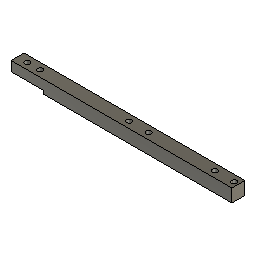
Horizontal_V11 (Autodesk Fusion 360 archive; units mm, degrees)
design "MainArm_Square"
description: .5"x.5"x8.5"
Autodesk Fusion 360 part; units mm, degrees
note: some values were not read from the file. Set by a fixed rule: the direction of a hole.
sketch "LeftEnd" plane through (0, 0, 0) normal (1, 0, 0) x (0, 1, 0) in component "MainArm_Square"
  line L0 (-6.35, -6.35) -> (6.35, -6.35)
  line L1 (6.35, -6.35) -> (6.35, 6.35)
  line L2 (6.35, 6.35) -> (-6.35, 6.35)
  line L3 (-6.35, 6.35) -> (-6.35, -6.35)
  line L4 (-6.35, -6.35) -> (6.35, 6.35) construction
  line L5 (6.35, -6.35) -> (-6.35, 6.35) construction
  dimension "d1" = 12.7
  dimension "d2" = 12.7
  constraint horizontal L0
  constraint perpendicular L0 L1
  constraint parallel L0 L2
  constraint parallel L1 L3
  constraint coincident L4 origin
  constraint coincident L5 origin
  measures "d1" distance of L1.end L2.end
  measures "d2" distance of L0.end L1.end
sketch "Top" plane through (0, 0, 0) normal (0, 0, 1) x (1, 0, 0) in component "MainArm_Square"
  line L0 (107.95, -6.35) -> (-107.95, -6.35)
  line L1 (-107.95, -6.35) -> (-107.95, 6.35)
  line L2 (-107.95, 6.35) -> (107.95, 6.35)
  line L3 (107.95, 6.35) -> (107.95, -6.35)
  line L4 (107.95, -6.35) -> (-107.95, 6.35) construction
  line L5 (-107.95, -6.35) -> (107.95, 6.35) construction
  circle A0 centre (104.013, 0) radius 2.4892
  circle A1 centre (84.963, 0) radius 2.4892
  circle A2 centre (-98.425, 0) radius 2.4892
  circle A3 centre (-85.725, 0) radius 2.4892
  line L6 (-76.073, 6.35) -> (-76.073, -6.35)
  circle A4 centre (1.143, 0) radius 2.4892
  circle A5 centre (20.193, 0) radius 2.4892
  dimension "d3" = 215.9
  dimension "d4" = 12.7
  dimension "d5" = 4.9784
  dimension "d6" = 4.9784
  dimension "d7" = 3.937
  dimension "d8" = 19.05
  dimension "d9" = 4.9784
  dimension "d10" = 4.9784
  dimension "d11" = 85.725
  dimension "d12" = 12.7
  dimension "d15" = 31.877
  dimension "d19" = 4.9784
  dimension "d20" = 4.9784
  dimension "d21" = 87.757
  dimension "d23" = 19.05
  constraint horizontal L0
  constraint perpendicular L0 L1
  constraint parallel L0 L2
  constraint parallel L1 L3
  constraint coincident L4 origin
  constraint coincident L5 origin
  constraint horizontal origin A0.centre
  constraint horizontal A0.centre A1.centre
  constraint horizontal origin A3.centre
  constraint horizontal A2.centre A3.centre
  constraint coincident L2 L6.start
  constraint coincident L0 L6.end
  constraint horizontal origin A4.centre
  constraint horizontal origin A5.centre
  measures "d3" distance of L1.end L2.end
  measures "d4" distance of L0.end L1.end
  measures "d5" diameter of A0
  measures "d6" diameter of A1
  measures "d7" distance of L3 A0.centre
  measures "d8" distance of A0.centre A1.centre
  measures "d9" diameter of A2
  measures "d10" diameter of A3
  measures "d11" distance of A3.centre origin
  measures "d12" distance of A2.centre A3.centre
  measures "d15" distance of L1 L6
  measures "d19" diameter of A4
  measures "d20" diameter of A5
  measures "d21" distance of L3 A5.centre
  measures "d23" distance of A4.centre A5.centre
extrude "Extrude1" add sketch "Top" along normal mid plane 12.7 in component "MainArm_Square"
extrude "Extrude2" cut sketch "Top" along normal blind 3.2614 from surface at -6.35 contours L0 L1 L2 L6 in component "MainArm_Square"
component "MainArm_Square" placed x (1, 0, 0) y (0, 1, 0) z (0, 0, 1) at (0, 0, 0)
equation "d5 = d6"
equation "d10 = d9"
equation "d19 = d6"
equation "d20 = d6"

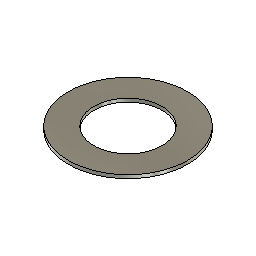
design "Washer_M4x7x0.2"
description: Bearing Washer: M4X7X0.2
Autodesk Fusion 360 part; units mm, degrees
sketch "Sketch1" plane through (0, 0, 0) normal (0, 0, 1) x (1, 0, 0)
  circle A0 centre (0, 0) radius 2
  circle A1 centre (0, 0) radius 3.5
  dimension "d1" = 4
  dimension "d2" = 7
  constraint coincident A0.centre A1.centre
  measures "d1" diameter of A0
  measures "d2" diameter of A1
extrude "Extrude1" add sketch "Sketch1" along normal blind 0.2

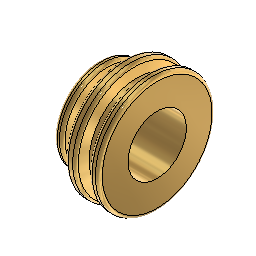
design "DoublePulley"
description: Pulley
Autodesk Fusion 360 part; units mm, degrees
sketch "Sketch2" plane through (0, 0, 0) normal (0, 0, 1) x (1, 0, 0)
  line L0 (-4.9843, -7.493) -> (-5.7409, -9.8217)
  line L1 (-4.9843, -7.493) -> (-3.6995, -7.493)
  line L2 (-3.6995, -7.493) -> (-2.0076, -12.7)
  line L3 (0.7769, -10.414) -> (0.0341, -12.7)
  line L4 (0.7769, -10.414) -> (2.4231, -10.414)
  line L5 (2.4231, -10.414) -> (3.1659, -12.7)
  circle A0 centre (1.6, -12.2784) radius 1.359 construction
  line L6 (3.1659, -12.7) -> (5.1858, -12.7)
  line L7 (-2.0076, -12.7) -> (0.0341, -12.7)
  circle A1 centre (-4.3419, -8.7519) radius 1 construction
  line L8 (-7.5142, -9.8217) -> (-7.5142, -6.35)
  line L9 (-7.5142, 0) -> (5, 0)
  line L10 (-7.5142, -6.35) -> (5.1858, -6.35)
  line L11 (5.1858, -12.7) -> (5.1858, -6.35)
  line L12 (-5.7409, -9.8217) -> (-7.5142, -9.8217)
  dimension "d142_1_1_1" = 12.7
  dimension "d145_1_1_1" = 108
  dimension "d146_1_1_1" = 108
  dimension "d147_1_1_1" = 1.6
  dimension "d150_1_1_1" = 10.414
  dimension "d152_1_1_1" = 12.2784
  dimension "d158_1_1_1" = 12.7
  dimension "d159_1_1_1" = 6.35
  dimension "d161_1_1_1" = 108
  dimension "d162_1_1_1" = 7.493
  dimension "d165_1_1_1" = 108
  dimension "d166_1_1_1" = 2
  dimension "d167_1_1_1" = 7.5142
  dimension "d169_1_1_1" = 9.8217
  dimension "d64_1_1" = 1.6462
  dimension "d65_1_1" = 2.5299
  dimension "d66_1_1" = 2.0418
  constraint perpendicular L10 L11
  constraint tangent L3 A0
  constraint tangent L5 A0
  constraint horizontal L7
  constraint horizontal L6
  constraint parallel L9 L10
  constraint horizontal L1
  constraint vertical L8
  constraint horizontal L12
  constraint tangent L2 A1
  constraint tangent L0 A1
  constraint collinear L6 L7
  constraint horizontal L4
  measures "d142_1_1_1" distance of origin L6
  measures "d145_1_1_1" angle of L3 L4
  measures "d146_1_1_1" angle of L4 L5
  measures "d147_1_1_1" horizontal distance of origin A0.centre
  measures "d150_1_1_1" distance of origin L4
  measures "d152_1_1_1" vertical distance of origin A0.centre
  measures "d158_1_1_1" distance of L10.end L8.end
  measures "d159_1_1_1" distance of origin L10
  measures "d161_1_1_1" angle of L2 L7
  measures "d162_1_1_1" distance of origin L1
  measures "d165_1_1_1" angle of L0 L1
  measures "d166_1_1_1" diameter of A1
  measures "d167_1_1_1" horizontal distance of origin L8.end
  measures "d169_1_1_1" distance of origin L12
  measures "d64_1_1" distance of L3.start L4.end
  measures "d65_1_1" distance of L0.start L8
  measures "d66_1_1" distance of L3.end L2.end
revolve "Revolve2" add sketch "Sketch2" angle 360 about axis through (-7.5142, 0, 0) along (1, 0, 0)
fillet "Fillet1" radius 0.75 6 edges at (-7.5142, -3.5517, -9.1571) (-5.7409, -3.5517, -9.1571) (-2.0076, -4.5925, -11.8406) (0.0341, -4.5925, -11.8406) (3.1659, -4.5925, -11.8406) (5.1858, -4.5925, -11.8406)
equation "d116_1 = 0.0000 in"
equation "d117_1 = 0.0000 in"
equation "d118_1 = 0.0000 in"
equation "d119_1 = 0.000 deg"
equation "d128_1 = 0.0000 in"
equation "d129_1 = 0.0000 in"
equation "d130_1 = 0.0000 in"
equation "d131_1 = 0.000 deg"

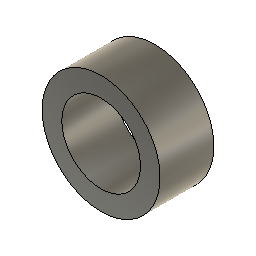
design "Spacer"
description: 1/4" X 3/8" X0.171"
Autodesk Fusion 360 part; units mm, degrees
sketch "Sketch1" plane through (0, 0, 0) normal (0, 1, 0) x (1, 0, 0)
  circle A0 centre (0, 0) radius 3.175
  circle A1 centre (0, 0) radius 4.7625
  dimension "d1" = 6.35
  dimension "d2" = 9.525
  constraint coincident A0.centre A1.centre
  constraint concentric A0 A1
  measures "d1" diameter of A0
  measures "d2" diameter of A1
extrude "Extrude1" add sketch "Sketch1" along normal blind 4.3434

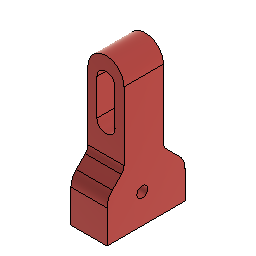
design "Tower"
Autodesk Fusion 360 part; units mm, degrees
sketch "Right" plane through (0, 0, 0) normal (1, 0, 0) x (0, 1, 0) in component "Tower"
  line L0 (0, 0) -> (0, 11.6117)
  line L1 (27.432, 9.9611) -> (27.432, 0)
  arc A0 (27.432, 9.9611) -> (25.5721, 14.4512) centre (21.082, 9.9611) ccw
  arc A1 (1.8541, 16.096) -> (0, 11.6117) centre (6.35, 11.6117) ccw
  arc A2 (5.0391, 19.281) -> (5.969, 21.526) centre (2.794, 21.526) ccw
  line L2 (5.0391, 19.281) -> (1.8541, 16.096)
  line L3 (20.7419, 19.2814) -> (25.5721, 14.4512)
  arc A3 (19.812, 21.5265) -> (20.7419, 19.2814) centre (22.987, 21.5265) ccw
  line L4 (19.812, 51.8592) -> (19.812, 21.5265)
  line L5 (19.812, 51.8592) -> (5.969, 51.8592)
  line L6 (5.969, 21.526) -> (5.969, 51.8592)
  line L7 (0, 0) -> (27.432, 0)
  circle A4 centre (12.3596, 10.3275) radius 1.8986
  line L8 (3.937, 0) -> (3.937, 12.7) construction
  line L9 (22.987, 0) -> (22.987, 12.7) construction
  circle A5 centre (12.3596, 10.3275) radius 12.7 construction
  dimension "d1" = 27.432
  dimension "d4" = 10.3275
  dimension "d5" = 6.35
  dimension "d6" = 6.8309
  dimension "d7" = 3.175
  dimension "d8" = 3.175
  dimension "d9" = 6.35
  dimension "d11" = 30.3327
  dimension "d13" = 13.843
  dimension "d14" = 9.9611
  dimension "d16" = 45
  dimension "d17" = 45
  dimension "d19" = 3.937
  dimension "d20" = 19.05
  dimension "d21" = 4.445
  dimension "d22" = 3.7973
  dimension "d23" = 12.3596
  dimension "d24" = 25.5721
  dimension "d25" = 14.4512
  dimension "d26" = 21.5265
  dimension "d28" = 12.7
  dimension "d29" = 12.7
  dimension "d46" = 16.096
  dimension "d47" = 1.8541
  dimension "d48" = 25.4
  constraint tangent A2 L6
  constraint perpendicular L1 L7
  constraint vertical L6
  constraint horizontal L5
  constraint vertical L4
  constraint horizontal L7
  constraint vertical L0
  constraint coincident L0.start L7.start
  constraint coincident L7 L8.start
  constraint perpendicular L7 L8
  constraint coincident L7 L9.start
  constraint perpendicular L7 L9
  constraint tangent A3 L4
  constraint tangent L0 A1
  constraint tangent A2 L2
  constraint concentric A4 A5
  measures "d1" distance of L0.start L1.end
  measures "d4" vertical distance of L0.start A4.centre
  measures "d5" radius of A0
  measures "d6" distance of A0.end L3.start
  measures "d7" radius of A3
  measures "d8" radius of A2
  measures "d9" radius of A1
  measures "d11" distance of A3.start L4.start
  measures "d13" distance of L4.start L5.end
  measures "d14" distance of L1.start L1.end
  measures "d16" angle of L3 L7
  measures "d17" angle of L2 L7
  measures "d19" distance of L0 L8
  measures "d20" distance of L8 L9
  measures "d21" distance of L1 L9
  measures "d22" diameter of A4
  measures "d23" horizontal distance of L0.start A4.centre
  measures "d24" horizontal distance of L0.start A0.end
  measures "d25" vertical distance of L0.start A0.end
  measures "d26" vertical distance of L0.start A3.start
  measures "d28" distance of L8.start L8.end
  measures "d29" distance of L9.start L9.end
  measures "d46" vertical distance of L0.start A1.start
  measures "d47" horizontal distance of L0.start A1.start
  measures "d48" diameter of A5
extrude "Extrude1" add sketch "Right" along normal mid plane 12.7 in component "Tower"
sketch "Front" plane through (0, 0, 0) normal (0, 1, 0) x (1, 0, 0) in component "Tower"
  line L0 (3.175, -43.9217) -> (3.175, -31.2217)
  arc A0 (3.175, -31.2217) -> (-3.175, -31.2217) centre (0, -31.2217) ccw
  line L1 (-3.175, -31.2217) -> (-3.175, -43.9217)
  arc A1 (-3.175, -43.9217) -> (3.175, -43.9217) centre (0, -43.9217) ccw
  line L2 (0, -43.9217) -> (0, -31.2217) construction
  dimension "d32" = 6.35
  dimension "d33" = 31.2217
  dimension "d34" = 12.7
  dimension "d35" = 3.175
  constraint tangent L0 A0
  constraint tangent A0 L1
  constraint parallel L0 L1
  constraint tangent L1 A1
  constraint tangent L0 A1
  constraint vertical L2
  measures "d32" diameter of A0
  measures "d33" vertical distance of A0.centre origin
  measures "d34" distance of A1.centre A0.centre
  measures "d35" horizontal distance of origin A0.end
extrude "Extrude2" cut sketch "Front" along normal up to surface (19.812 mm away) in component "Tower"
sketch "Bottom" plane through (0, 0, 0) normal (0, 0, 1) x (1, 0, 0) in component "Tower"
  circle A0 centre (0, 3.937) radius 1.8986
  circle A1 centre (0, 22.987) radius 1.8986
  dimension "d38" = 19.05
  dimension "d39" = 3.7973
  dimension "d40" = 3.7973
  dimension "d41" = 3.937
  constraint vertical A0.centre origin
  constraint vertical A0.centre A1.centre
  measures "d38" distance of A0.centre A1.centre
  measures "d39" diameter of A1
  measures "d40" diameter of A0
  measures "d41" distance of origin A0.centre
hole "Hole1" at (0, 22.987, 0) at (0, 3.937, 0) direction (0, 0, 1) diameter 3.7973 depth 14.224 tip angle 118 in component "Tower"
fillet "Fillet1" radius 6.35 2 edges at (-6.35, 12.8905, 51.8592) (6.35, 12.8905, 51.8592) in component "Tower"
component "Tower" placed x (1, 0, 0) y (0, 1, 0) z (0, 0, 1) at (0, 0, 0)
equation "d39 = d40"

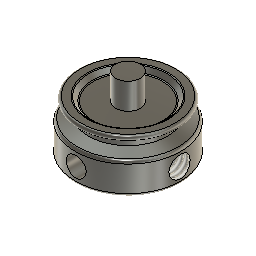
design "Horizontal_CutterHead"
description: .125" cutters MF104ZZ bearings 2mm belt
Autodesk Fusion 360 part; units mm, degrees
sketch "Sketch1" plane through (0, 0, 0) normal (0, 1, 0) x (1, 0, 0)
  line L0 (0, 6.7947) -> (0, -9.0975)
  line L1 (2, -9.0975) -> (0, -9.0975)
  line L2 (2, -4.8975) -> (2, -9.0975)
  line L3 (7.621, -5.6475) -> (6.5104, -5.6475)
  line L4 (7.7395, -4.9005) -> (6.35, -4.4484)
  line L5 (8.495, -2.4737) -> (6.35, -3.1716)
  circle A0 centre (7.62, -3.81) radius 1 construction
  line L6 (8.495, 2.5407) -> (2, 2.5407)
  line L7 (8.495, 2.5407) -> (8.495, -2.4737)
  line L8 (2, 6.7947) -> (2, 2.5407)
  line L9 (2, 6.7947) -> (0, 6.7947)
  circle A1 centre (0, 0) radius 1.7272
  circle A2 centre (0, 0) radius 2.0828 construction
  circle A3 centre (0, 0) radius 1.5875
  line L10 (6.35, -4.4484) -> (6.35, -3.1716)
  arc A4 (7.621, -5.6475) -> (7.7395, -4.9005) centre (7.621, -5.2646) ccw
  circle A5 centre (0, 0) radius 12.7 construction
  circle A6 centre (0, 0) radius 11.1125 construction
  line L11 (5.55, -4.8975) -> (2, -4.8975)
  arc A7 (5.7296, -4.9719) -> (5.55, -4.8975) centre (5.55, -5.1515) ccw
  line L12 (8.495, -2.4737) -> (0, -2.4737) construction
  line L13 (6.3308, -5.5731) -> (5.7296, -4.9719)
  arc A8 (6.3308, -5.5731) -> (6.5104, -5.6475) centre (6.5104, -5.3935) ccw
  dimension "d30" = 2
  dimension "d50" = 0
  dimension "d51" = 0
  dimension "d52" = 0
  dimension "d53" = 0
  dimension "d62" = 0
  dimension "d63" = 0
  dimension "d64" = 0
  dimension "d65" = 0
  dimension "d93" = 3.4544
  dimension "d94" = 4.1656
  dimension "d96" = 3.175
  dimension "d98" = 6.7947
  dimension "d99" = 2
  dimension "d101" = 2
  dimension "d102" = 8.495
  dimension "d110" = 3.81
  dimension "d111" = 7.62
  dimension "d114" = 6.35
  dimension "d116" = 108.025
  dimension "d117" = 108.025
  dimension "d121" = 5.0144
  dimension "d122" = 0.3829
  dimension "d153" = 25.4
  dimension "d154" = 22.225
  dimension "d170" = 0.75
  dimension "d180" = 0
  dimension "d181" = 0
  dimension "d182" = 0
  dimension "d183" = 0
  dimension "d224" = 4.2
  dimension "d227" = 15.8922
  dimension "d1" = 135
  dimension "d2" = 0.254
  dimension "d3" = 0.254
  dimension "d4" = 5.7296
  constraint tangent L4 A0
  constraint tangent L5 A0
  constraint vertical L8
  constraint perpendicular L0 L9
  constraint coincident A1.centre A2.centre
  constraint vertical L0
  constraint horizontal L1
  constraint vertical L10
  constraint tangent L4 A4
  constraint tangent L3 A4
  constraint horizontal L3
  constraint vertical L2
  constraint vertical L7
  constraint concentric A1 A5
  constraint concentric A3 A6
  constraint tangent L11 A7
  constraint coincident L0 L12.end
  constraint perpendicular L0 L12
  constraint horizontal L6
  constraint coincident L0 A1.centre
  constraint tangent A7 L13
  constraint tangent L13 A8
  constraint tangent L3 A8
  measures "d30" diameter of A0
  measures "d93" diameter of A1
  measures "d94" diameter of A2
  measures "d96" diameter of A3
  measures "d98" distance of L9 A1.centre
  measures "d99" distance of L8.start L0.start
  measures "d101" distance of L0.end L1.start
  measures "d102" distance of A1.centre L7
  measures "d110" vertical distance of A0.centre A1.centre
  measures "d111" horizontal distance of A0.centre A1.centre
  measures "d114" distance of A1.centre L10
  measures "d116" angle of L5 L10
  measures "d117" angle of L4 L10
  measures "d121" distance of L6.start L5.start
  measures "d153" diameter of A5
  measures "d154" diameter of A6
  measures "d170" distance of L3 L11
  measures "d224" distance of L1.start L2.start
  measures "d227" distance of L0.end L0.start
  measures "d1" angle of L3 L13
  measures "d2" radius of A7
  measures "d3" radius of A8
  measures "d4" horizontal distance of A1.centre A7.start
revolve "Revolve3" add sketch "Sketch1" angle 360 about axis through (0, 0, -6.7947) along (0, 0, 1) contours L0 L1 L2 L3 L4 L5 L6 L7 L8 L9 A1 L10 A4 L11 A7 L13 A8 | L0 A1 A3 | L0 A3 picked at (0.0819, -1.6748) picked at (0.3465, 0.3999)
extrude "Extrude5" cut sketch "Sketch1" along normal mid plane 28.2346 contours L0 A1 A3 | L0 A1 A3 | L0 A3 | L0 A3
move_face "MoveFace2" to x (0, 1, 0) y (-1, 0, 0) z (0, 0, 1) at (0.0002, -0.0002, 0) 1 faces at (0.425, -2.8249, -1.6741)
extrude "Extrude6" cut sketch "Sketch1" along normal mid plane 24.5974 contours L0 A3 | L0 A3
thread "Thread2" "ANSI Unified Screw Threads 0.164(#8) 8-32 UNC 3B" major diameter 4.1656 minor diameter 3.4163 pitch 0.7937 angle 60 resizes the face on face at (0.008, -0.4552, 1.6662)
fillet "Fillet2" radius 0.508 2 edges at (-7.9201, -3.0719, 2.4737) (-7.9201, -3.0719, -2.5407)
equation "d101 = d99"
equation "d117 = d116"
equation "d3 = d2"
